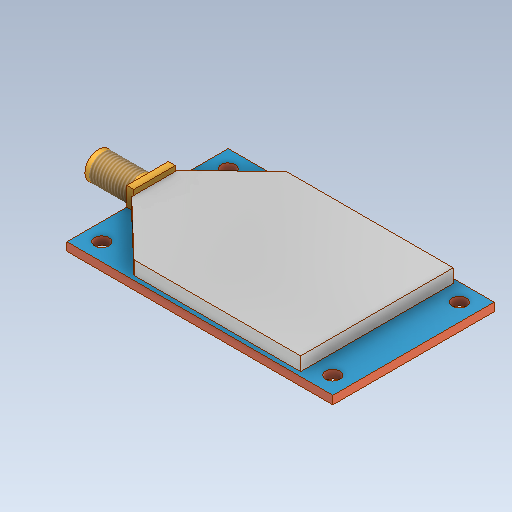
# Autodesk Inventor part: XT09-SI
Saved by Autodesk Inventor 2020.2 (Build 242310000, 310)
## iProperties
Created: 2020-04-10
Part Number: XT09-SI
Material: Phenolic Resin
Document SubType Name: Modeling
Designer: agmlego
Mass: 13.4655 g
Surface Area: 57.1409 cm^2
Volume: 9.75758 cm^3
Density: 1.38 g/cm^3
Appearance: Smooth - Light Orange
Author: agmlego
Autodesk Inventor part; units mm, degrees
ref_plane "YZ Plane" through (0, 0, 0) normal (1, 0, 0) x (0, 1, 0)
ref_plane "XZ Plane" through (0, 0, 0) normal (0, 1, 0) x (-1, 0, 0)
ref_plane "XY Plane" through (0, 0, 0) normal (0, 0, 1) x (1, 0, 0)
sketch "Sketch1" plane through (0, 0, 0) normal (0, 1, 0) x (-1, 0, 0)
  line L0 (0, 0) -> (61, 0)
  line L1 (61, 0) -> (61, -37)
  line L2 (61, -37) -> (0, -37)
  line L3 (0, -37) -> (0, 0)
  dimension "d0" = 61
  dimension "d1" = 37
  constraints: 8 end point, 2 parallel, 1 horizontal, 1 perpendicular
  measures "d0" distance of L0.start L0.end
  measures "d1" distance of L2.end L0.start
extrude "PCB" add sketch "Sketch1" along normal blind 1.9
sketch "Sketch2" plane through (0, 1.9, 0) normal (0, 1, 0) x (1, 0, 0)
  circle A0 centre (-57, 4) radius 4 construction
  circle A1 centre (-57, 33) radius 4 construction
  circle A2 centre (-4, 33) radius 4 construction
  circle A3 centre (-4, 4) radius 4 construction
  line L0 (-61, 37) -> (-61, 0) construction
  line L1 (-61, 0) -> (0, 0) construction
  line L2 (0, 37) -> (-61, 37) construction
  line L3 (0, 0) -> (0, 37) construction
  dimension "d4" = 8
  constraints: 8 tangent, 4 centre point, 4 coincident, 3 equal radius
  measures "d4" diameter of A0
hole "Mounting" at (-57, 1.9, -4) at (-57, 1.9, -33) at (-4, 1.9, -33) at (-4, 1.9, -4) direction (0, -1, 0) diameter 3.3 end through all start extended yes
sketch "Sketch3" plane through (0, 1.9, 0) normal (0, 1, 0) x (1, 0, 0)
  line L0 (-59.4, 13.25) -> (-46.6, 1)
  line L1 (-46.6, 1) -> (-8.4, 1)
  line L2 (-8.4, 1) -> (-8.4, 36)
  line L3 (-8.4, 36) -> (-46.6, 36)
  line L4 (-46.6, 36) -> (-59.4, 23.75)
  line L5 (-59.4, 23.75) -> (-59.4, 13.25)
  line L6 (-59.4, 18.5) -> (-8.4, 18.5) construction
  line L7 (-61, 37) -> (-61, 0) projected
  point P0 (0, 0)
  point P1 (-61, 18.5)
  dimension "d12" = 35
  dimension "d13" = 10.5
  dimension "d14" = 51
  dimension "d15" = 38.2
  dimension "d18" = 1.6
  constraints: 15 end point, 4 perpendicular, 3 midpoint, 2 equal length, 1 horizontal, 1 point on line
  measures "d12" distance of L1.end L2.end
  measures "d13" distance of L4.end L0.start
  measures "d14" distance of L6.start L6.end
  measures "d15" distance of L0.end L1.end
  measures "d18" distance between parallel lines of L7 L5
extrude "RF Can" add sketch "Sketch3" along normal blind 3.12
sketch "Sketch4" plane through (-59.4, 1.9, -23.75) normal (-1, 0, 0) x (0, 0, 1)
  line L0 (0.5, 4.3) -> (10, 4.3)
  line L1 (10, 4.3) -> (10, -3.6)
  line L2 (10, -3.6) -> (0.5, -3.6)
  line L3 (0.5, -3.6) -> (0.5, 4.3)
  line L4 (-13.25, 0) -> (23.75, 0) projected
  line L5 (5.25, 4.3) -> (5.25, 0) construction
  line L6 (10.5, 0) -> (0, 0) construction
  point P0 (23.75, -1.9)
  dimension "d19" = 9.5
  dimension "d20" = 7.9
  dimension "d21" = 4.3
  constraints: 10 end point, 2 midpoint, 2 parallel, 2 perpendicular, 1 horizontal
  measures "d19" distance of L0.start L0.end
  measures "d20" distance of L2.end L0.start
  measures "d21" distance between parallel lines of L4 L0
extrude "Extrusion3" add sketch "Sketch4" along normal blind 1.61
sketch "Sketch5" plane through (-59.4, 1.9, -23.75) normal (1, 0, 0) x (0, 0, -1)
  line L0 (-10, -3.6) -> (-10, -1.9) projected
  line L1 (-10, -3.6) -> (-8.9, -3.6)
  line L2 (-8.9, -3.6) -> (-8.9, -1.9)
  line L3 (-8.9, -1.9) -> (-10, -1.9)
  line L4 (-10, -1.9) -> (-10, -3.6)
  line L5 (-0.5, -1.9) -> (-0.5, -3.6) projected
  line L6 (-10, -1.9) -> (-0.5, -1.9) projected
  line L7 (-0.5, -3.6) -> (-1.6, -3.6)
  line L8 (-1.6, -3.6) -> (-1.6, -1.9)
  line L9 (-1.6, -1.9) -> (-0.5, -1.9)
  line L10 (-0.5, -1.9) -> (-0.5, -3.6)
  point P0 (-23.75, -1.9)
  dimension "d24" = 1.1
  constraints: 16 end point, 4 parallel, 2 collinear, 2 horizontal, 2 perpendicular, 1 point on line
  measures "d24" distance of L0.start L1.end
extrude "Extrusion4" add sketch "Sketch5" along normal blind 4.6
sketch "Sketch6" plane through (-61.01, 1.9, -23.75) normal (-1, 0, 0) x (0, 0, 1)
  circle A0 centre (5.25, 0.35) radius 3.125
  line L0 (10, 4.3) -> (0.5, 4.3) construction
  line L1 (5.25, 4.3) -> (5.25, -3.6) construction
  line L2 (1.6, -3.6) -> (8.9, -3.6) construction
  point P0 (23.75, -1.9)
  point P1 (5.25, 0.35)
  dimension "d27" = 6.25
  constraints: 3 midpoint, 2 end point, 1 centre point, 1 coincident
  measures "d27" diameter of A0
extrude "Extrusion5" add sketch "Sketch6" along normal blind 11.25
thread "Thread1" size "1/4-36 UNS" class "2A" standard "ANSI Unified Screw Threads" length 8.75 offset 1
body "Solid1"
